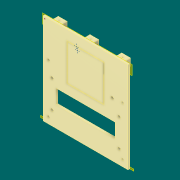
# Autodesk Inventor part: Front
Saved by Autodesk Inventor 2019 (Build 230136000, 136)
## iProperties
Created: 2025-01-01
Part Number: Front
Material: Nylon 6/6
Document SubType Name: Modeling
Designer: Familia CS
Density: 1.13 g/cm^3
Appearance: Nylon 6
Author: Familia CS
Autodesk Inventor part; units mm, degrees
ref_plane "YZ Plane" through (0, 0, 0) normal (1, 0, 0) x (0, 1, 0)
ref_plane "XZ Plane" through (0, 0, 0) normal (0, 1, 0) x (-1, 0, 0)
ref_plane "XY Plane" through (0, 0, 0) normal (0, 0, 1) x (1, 0, 0)
ref_plane "Work Plane1" through (0, 0, 0) normal (0, 0, 1) x (1, 0, 0)
sketch "Sketch1" plane through (0, 0, 0) normal (0, 0, 1) x (1, 0, 0)
  line L0 (5, 0) -> (86, 0) projected
  line L1 (86, -8) -> (86, 0) projected
  line L2 (5, 0) -> (5, -8) projected
  line L3 (43, 0) -> (43, -8) projected
  line L4 (53, -8) -> (53, 0) projected
  line L5 (86, 0) -> (76, 0)
  line L6 (76, 0) -> (76, -8)
  line L7 (76, -8) -> (86, -8)
  line L8 (86, -8) -> (86, 0)
  line L9 (5, 0) -> (15, 0)
  line L10 (15, 0) -> (15, -8)
  line L11 (15, -8) -> (5, -8)
  line L12 (5, -8) -> (5, 0)
  point P0 (0, 0)
  dimension "d0" = 10
  dimension "d1" = 8
  dimension "d3" = 10
  dimension "d4" = 8
  constraints: 16 end point, 4 parallel, 2 horizontal, 2 perpendicular
  measures "d0" distance of L7.end L6.end
  measures "d1" distance of L6.end L5.end
  measures "d3" distance of L10.end L11.end
  measures "d4" distance of L9.end L10.end
extrude "Extrusion1" add sketch "Sketch1" against normal blind 8
sketch "Sketch2" plane through (0, 0, 0) normal (0, 0, 1) x (1, 0, 0)
  line L0 (15, 0) -> (15, -8) projected
  line L1 (76, -8) -> (76, 0) projected
  line L2 (15, -8) -> (76, -8)
  line L3 (45.5, -8) -> (40.5, -8)
  line L4 (40.5, -8) -> (40.5, 0)
  line L5 (40.5, 0) -> (50.5, 0)
  line L6 (50.5, 0) -> (50.5, -8)
  point P0 (0, 0)
  dimension "d7" = 5
  dimension "d8" = 10
  constraints: 10 end point, 3 perpendicular, 2 point on line, 1 horizontal, 1 midpoint
  measures "d7" distance of L3.start L3.end
  measures "d8" distance of L4.end L5.end
extrude "Extrusion2" add sketch "Sketch2" against normal blind 8
sketch "Sketch3" plane through (76, -8, 0) normal (0, -1, 0) x (1, 0, 0)
  line L0 (10, -8) -> (0, -8) projected
  circle A0 centre (5, -4) radius 0.75
  line L1 (-25.5, -8) -> (-35.5, -8) projected
  circle A1 centre (-30.5, -4) radius 0.75
  line L2 (-61, -8) -> (-71, -8) projected
  circle A2 centre (-66, -4) radius 0.75
  point P0 (-76, 0)
  dimension "d12" = 1.5
  dimension "d14" = 1.5
  dimension "d16" = 1.5
  constraints: 3 centre point
  measures "d12" diameter of A0
  measures "d14" diameter of A1
  measures "d16" diameter of A2
extrude "Extrusion3" cut sketch "Sketch3" against normal blind 8
ref_plane "Work Plane2" through (93, -98, 0) normal (0, 0, 1) x (-1, 0, 0)
sketch "Sketch4" plane through (93, -98, 0) normal (0, 0, 1) x (-1, 0, 0)
  line L0 (10, 0) -> (10, -10) projected
  line L1 (85, 0) -> (85, -10) projected
  line L2 (95, 0) -> (0, 0) projected
  line L3 (10, 0) -> (20, 0)
  line L4 (20, 0) -> (20, -10)
  line L5 (20, -10) -> (10, -10)
  line L6 (10, -10) -> (10, 0)
  line L7 (85, -10) -> (75, -10)
  line L8 (75, -10) -> (75, 0)
  line L9 (75, 0) -> (85, 0)
  line L10 (85, 0) -> (85, -10)
  line L11 (75, 0) -> (20, 0)
  line L12 (47.5, -10) -> (52.5, -10)
  line L13 (52.5, -10) -> (52.5, 0)
  line L14 (52.5, 0) -> (42.5, 0)
  line L15 (42.5, 0) -> (42.5, -10)
  line L16 (42.5, -10) -> (47.5, -10)
  point P0 (93, -98)
  dimension "d19" = 10
  dimension "d20" = 10
  dimension "d21" = 10
  dimension "d22" = 10
  dimension "d24" = 5
  dimension "d25" = 10
  dimension "d26" = 10
  dimension "d27" = 10
  constraints: 28 end point, 4 parallel, 3 horizontal, 3 point on line, 2 perpendicular
  measures "d19" distance of L4.end L5.end
  measures "d20" distance of L3.end L4.end
  measures "d21" distance of L8.end L9.end
  measures "d22" distance of L7.end L8.end
  measures "d24" distance of L12.start L12.end
  measures "d25" distance of L12.end L13.end
  measures "d26" distance of L13.end L14.end
  measures "d27" distance of L14.end L15.end
extrude "Extrusion4" add sketch "Sketch4" against normal blind 8
sketch "Sketch5" plane through (73, -88, 0) normal (0, 1, 0) x (1, 0, 0)
  line L0 (10, 0) -> (0, 0) projected
  circle A0 centre (5, 4) radius 0.75
  line L1 (-22.5, 0) -> (-32.5, 0) projected
  circle A1 centre (-27.5, 4) radius 0.75
  line L2 (-55, 0) -> (-65, 0) projected
  circle A2 centre (-60, 4) radius 0.75
  point P0 (-73, 0)
  dimension "d31" = 1.5
  dimension "d33" = 1.5
  dimension "d35" = 1.5
  constraints: 3 centre point
  measures "d31" diameter of A0
  measures "d33" diameter of A1
  measures "d35" diameter of A2
extrude "Extrusion5" cut sketch "Sketch5" against normal blind 10
sketch "Sketch6" plane through (93, -98, 0) normal (0, 0, 1) x (1, 0, 0)
  line L0 (0, 0) -> (0, -2) projected
  line L1 (-93, 100) -> (-95, 100) projected
  line L2 (-95, 100) -> (0, 100)
  line L3 (0, 100) -> (0, -2)
  line L4 (0, -2) -> (-95, -2)
  line L5 (-95, -2) -> (-95, 100)
  circle A0 centre (-6, 50) radius 0.75 projected
  circle A1 centre (-6, 5) radius 0.75 projected
  circle A2 centre (-89, 5) radius 0.75 projected
  circle A3 centre (-89, 50) radius 0.75 projected
  point P0 (-93, 98)
  constraints: 8 end point, 2 parallel, 1 horizontal, 1 perpendicular
extrude "Extrusion6" add sketch "Sketch6" along normal blind 2
sketch "Sketch7" plane through (93, -98, 0) normal (0, 0, -1) x (-1, 0, 0)
  line L0 (42.5, 90) -> (52.5, 90) projected
  line L1 (47.5, 84) -> (80.5, 84)
  line L2 (80.5, 84) -> (80.5, 68)
  line L3 (80.5, 68) -> (14.5, 68)
  line L4 (14.5, 68) -> (14.5, 84)
  line L5 (14.5, 84) -> (47.5, 84)
  point P0 (93, 98)
  dimension "d41" = 33
  dimension "d42" = 16
  dimension "d43" = 66
  constraints: 10 end point, 4 perpendicular, 1 horizontal, 1 point on line
  measures "d41" distance of L1.start L1.end
  measures "d42" distance of L1.end L2.end
  measures "d43" distance of L2.end L3.end
extrude "Extrusion7" cut sketch "Sketch7" against normal blind 2
sketch "Sketch8" plane through (93, -98, 0) normal (0, 0, -1) x (-1, 0, 0)
  line L0 (14.5, 84) -> (80.5, 84) projected
  circle A0 centre (85.1, 86.9) radius 1.375
  circle A1 centre (9.9, 86.9) radius 1.375
  line L1 (80.5, 68) -> (14.5, 68) projected
  circle A2 centre (9.9, 65.1) radius 1.375
  circle A3 centre (85.1, 65.1) radius 1.375
  point P0 (93, 98)
  dimension "d50" = 2.75
  dimension "d54" = 2.75
  dimension "d61" = 2.75
  dimension "d64" = 2.75
  constraints: 4 centre point
  measures "d50" diameter of A0
  measures "d54" diameter of A1
  measures "d61" diameter of A2
  measures "d64" diameter of A3
extrude "Extrusion8" cut sketch "Sketch8" against normal blind 2
sketch "Sketch9" plane through (93, -98, 2) normal (0, 0, 1) x (1, 0, 0)
  line L0 (-88, 88.797) -> (-7.6952, 88.797)
  line L1 (-7.6952, 88.797) -> (-7.6952, 63.1475)
  line L2 (-7.6952, 63.1475) -> (-88, 63.1475)
  line L3 (-88, 63.1475) -> (-88, 88.797)
  point P0 (-93, 98)
  constraints: 8 end point, 2 parallel, 1 horizontal, 1 perpendicular
extrude "Extrusion9" add sketch "Sketch9" against normal blind 2
sketch "Sketch10" plane through (93, -98, 0) normal (0, 0, -1) x (-1, 0, 0)
  line L0 (42.5, 10) -> (52.5, 10) projected
  line L1 (47.5, 16) -> (14.5, 16)
  line L2 (14.5, 16) -> (14.5, 32)
  line L3 (14.5, 32) -> (80.5, 32)
  line L4 (80.5, 32) -> (80.5, 16)
  line L5 (80.5, 16) -> (47.5, 16)
  circle A0 centre (9.9, 13.1) radius 1.375
  circle A1 centre (85.1, 13.1) radius 1.375
  line L6 (47.5, 32) -> (47.5, 37.4)
  circle A2 centre (85.1, 34.9) radius 1.375
  circle A3 centre (9.9, 34.9) radius 1.375
  point P0 (93, 98)
  dimension "d70" = 33
  dimension "d71" = 16
  dimension "d72" = 66
  dimension "d73" = 16
  dimension "d74" = 33
  dimension "d80" = 2.75
  dimension "d83" = 2.75
  dimension "d84" = 5.4
  dimension "d89" = 2.75
  dimension "d92" = 2.75
  constraints: 12 end point, 4 centre point, 2 perpendicular, 1 midpoint, 1 point on line, 1 vertical
  measures "d70" distance of L1.start L1.end
  measures "d71" distance of L1.end L2.end
  measures "d72" distance of L2.end L3.end
  measures "d73" distance of L3.end L4.end
  measures "d74" distance of L4.end L1.start
  measures "d80" diameter of A0
  measures "d83" diameter of A1
  measures "d84" distance of L6.start L6.end
  measures "d89" diameter of A2
  measures "d92" diameter of A3
extrude "Extrusion10" cut sketch "Sketch10" against normal blind 2
sketch "Sketch11" plane through (93, -98, 0) normal (0, 0, -1) x (-1, 0, 0)
  circle A0 centre (85.1, 13.1) radius 1.375 projected
  line L0 (8.0573, 36.8158) -> (87.4686, 36.8158)
  line L1 (87.4686, 36.8158) -> (87.4686, 10.2199)
  line L2 (87.4686, 10.2199) -> (8.0573, 10.2199)
  line L3 (8.0573, 10.2199) -> (8.0573, 36.8158)
  point P0 (93, 98)
  constraints: 8 end point, 2 parallel, 1 horizontal, 1 perpendicular
extrude "Extrusion11" add sketch "Sketch11" against normal blind 2
sketch "Sketch12" plane through (93, -98, 0) normal (0, 0, -1) x (-1, 0, 0)
  line L0 (82.8776, 15.0849) -> (86.9969, 15.0849)
  line L1 (86.9969, 15.0849) -> (86.9969, 11.175)
  line L2 (86.9969, 11.175) -> (82.8776, 11.175)
  line L3 (82.8776, 11.175) -> (82.8776, 15.0849)
  point P0 (93, 98)
  constraints: 8 end point, 2 parallel, 1 horizontal, 1 perpendicular
extrude "Extrusion12" add sketch "Sketch12" against normal blind 2
sketch "Sketch13" plane through (93, -98, 0) normal (0, 0, -1) x (-1, 0, 0)
  line L0 (42.5, 10) -> (52.5, 10) projected
  circle A0 centre (85.1, 22.5) radius 2.75
  point P0 (93, 98)
  dimension "d104" = 5.5
  constraints: 1 centre point
  measures "d104" diameter of A0
extrude "Extrusion13" cut sketch "Sketch13" against normal blind 2
sketch "Sketch14" plane through (93, -98, 2) normal (0, 0, 1) x (1, 0, 0)
  line L0 (-88.4753, 26.414) -> (-81.2801, 26.414)
  line L1 (-81.2801, 26.414) -> (-81.2801, 18.3554)
  line L2 (-81.2801, 18.3554) -> (-88.4753, 18.3554)
  line L3 (-88.4753, 18.3554) -> (-88.4753, 26.414)
  point P0 (-93, 98)
  constraints: 8 end point, 2 parallel, 1 horizontal, 1 perpendicular
extrude "Extrusion14" add sketch "Sketch14" against normal blind 2
sketch "Sketch15" plane through (93, -98, 2) normal (0, 0, 1) x (1, 0, 0)
  point P0 (-93, 98)
sketch "Sketch16" plane through (93, -98, 0) normal (0, 0, -1) x (-1, 0, 0)
  line L0 (52.5, 90) -> (42.5, 90) projected
  circle A0 centre (9.9, 81.5) radius 1.5
  point P0 (93, 98)
  dimension "d118" = 3
  constraints: 1 centre point
  measures "d118" diameter of A0
extrude "Extrusion15" cut sketch "Sketch16" against normal blind 2
sketch "Sketch17" plane through (93, -98, 0) normal (0, 0, -1) x (-1, 0, 0)
  line L0 (7.2985, 84.1851) -> (12.7093, 84.1851)
  line L1 (12.7093, 84.1851) -> (12.7093, 78.544)
  line L2 (12.7093, 78.544) -> (7.2985, 78.544)
  line L3 (7.2985, 78.544) -> (7.2985, 84.1851)
  point P0 (93, 98)
  constraints: 8 end point, 2 parallel, 1 horizontal, 1 perpendicular
extrude "Extrusion16" add sketch "Sketch17" against normal blind 2
sketch "Sketch18" plane through (93, -98, 0) normal (0, 0, -1) x (-1, 0, 0)
  line L0 (42.5, 10) -> (52.5, 10) projected
  circle A0 centre (85.1, 18.5) radius 1.5
  point P0 (93, 98)
  dimension "d127" = 3
  constraints: 1 centre point
  measures "d127" diameter of A0
extrude "Extrusion17" cut sketch "Sketch18" against normal blind 2
sketch "Sketch19" plane through (93, -98, 0) normal (0, 0, -1) x (-1, 0, 0)
  line L0 (42.5, 10) -> (52.5, 10) projected
  circle A0 centre (9.9, 18.5) radius 1.5
  point P0 (93, 98)
  dimension "d134" = 3
  constraints: 1 centre point
  measures "d134" diameter of A0
extrude "Extrusion18" cut sketch "Sketch19" against normal blind 2
sketch "Sketch20" plane through (93, -98, 0) normal (0, 0, -1) x (-1, 0, 0)
  line L0 (6.951, 21.791) -> (88.5357, 21.791)
  line L1 (88.5357, 21.791) -> (88.5357, 14.1465)
  line L2 (88.5357, 14.1465) -> (6.951, 14.1465)
  line L3 (6.951, 14.1465) -> (6.951, 21.791)
  point P0 (93, 98)
  constraints: 8 end point, 2 parallel, 1 horizontal, 1 perpendicular
extrude "Extrusion19" add sketch "Sketch20" against normal blind 2
sketch "Sketch21" plane through (93, -98, 0) normal (0, 0, -1) x (-1, 0, 0)
  line L0 (42.5, 10) -> (52.5, 10) projected
  circle A0 centre (85.1, 13.5) radius 1.5
  circle A1 centre (9.9, 13.5) radius 1.5
  line L1 (47.5, 21) -> (80.5, 21)
  line L2 (80.5, 21) -> (80.5, 37)
  line L3 (80.5, 37) -> (14.5, 37)
  line L4 (14.5, 37) -> (14.5, 21)
  line L5 (14.5, 21) -> (47.5, 21)
  circle A2 centre (9.9, 44.5) radius 1.5
  circle A3 centre (85.1, 44.5) radius 1.5
  point P0 (93, 98)
  dimension "d143" = 3
  dimension "d147" = 3
  dimension "d150" = 33
  dimension "d151" = 16
  dimension "d152" = 66
  dimension "d157" = 3
  dimension "d161" = 3
  constraints: 10 end point, 4 centre point, 3 perpendicular, 1 horizontal, 1 vertical
  measures "d143" diameter of A0
  measures "d147" diameter of A1
  measures "d150" distance of L1.start L1.end
  measures "d151" distance of L1.end L2.end
  measures "d152" distance of L2.end L3.end
  measures "d157" diameter of A2
  measures "d161" diameter of A3
extrude "Extrusion20" cut sketch "Sketch21" against normal blind 2
sketch "Sketch22" plane through (93, -98, 0) normal (0, 0, -1) x (-1, 0, 0)
  line L0 (88.1, 50.9663) -> (90.0333, 50.9663)
  line L1 (90.0333, 50.9663) -> (90.0333, 48.9675)
  line L2 (90.0333, 48.9675) -> (88.1, 48.9675)
  line L3 (88.1, 48.9675) -> (88.1, 50.9663)
  line L4 (5.046, 50.7936) -> (6.9554, 50.7936)
  line L5 (6.9554, 50.7936) -> (6.9554, 48.9675)
  line L6 (6.9554, 48.9675) -> (5.046, 48.9675)
  line L7 (5.046, 48.9675) -> (5.046, 50.7936)
  point P0 (93, 98)
  constraints: 16 end point, 4 parallel, 2 horizontal, 2 perpendicular, 1 point on line
extrude "Extrusion21" add sketch "Sketch22" against normal blind 2
sketch "Sketch23" plane through (93, -98, 2) normal (0, 0, 1) x (1, 0, 0)
  point P0 (-93, 98)
  point P1 (-57.8, 88.8806)
  point P2 (-56.6, 85.3806)
  constraints: 2 other
sketch "Sketch24" plane through (93, -98, 2) normal (0, 0, 1) x (1, 0, 0)
  circle A0 centre (-89, 60) radius 0.75 projected
  point P0 (-93, 98)
extrude "Extrusion22" cut sketch "Sketch24" against normal blind 2
sketch "Sketch25" plane through (93, -98, 2) normal (0, 0, 1) x (1, 0, 0)
  circle A0 centre (-89, 60) radius 0.75 projected
  circle A1 centre (-89, 60) radius 1.25
  point P0 (-93, 98)
  dimension "d168" = 2.5
  constraints: 1 centre point, 1 coincident
  measures "d168" diameter of A1
extrude "Extrusion23" cut sketch "Sketch25" against normal blind 2
sketch "Sketch26" plane through (93, -98, 2) normal (0, 0, 1) x (1, 0, 0)
  circle A0 centre (-89, 5) radius 0.75 projected
  circle A1 centre (-89, 5) radius 1.25
  circle A2 centre (-6, 5) radius 0.75 projected
  circle A3 centre (-6, 5) radius 1.25
  point P0 (-93, 98)
  dimension "d171" = 2.5
  dimension "d172" = 2.5
  constraints: 2 centre point, 2 coincident
  measures "d171" diameter of A1
  measures "d172" diameter of A3
extrude "Extrusion24" cut sketch "Sketch26" against normal blind 2 contours A0 | A1 | A3
sketch "Sketch27" plane through (93, -98, 2) normal (0, 0, 1) x (1, 0, 0)
  point P0 (-93, 98)
sketch "Sketch28" plane through (93, -98, 2) normal (0, 0, 1) x (1, 0, 0)
  circle A0 centre (-6, 60) radius 0.75 projected
  circle A1 centre (-6, 60) radius 1.25
  point P0 (-93, 98)
  dimension "d175" = 2.5
  constraints: 1 centre point, 1 coincident
  measures "d175" diameter of A1
extrude "Extrusion25" cut sketch "Sketch28" against normal blind 2 contours A0 | A1
sketch "Sketch29" plane through (93, -98, 2) normal (0, 0, 1) x (1, 0, 0)
  circle A0 centre (-17.6001, 58.9999) radius 1.525 projected
  point P0 (-93, 98)
extrude "Extrusion26" cut sketch "Sketch29" against normal blind 2
sketch "Sketch30" plane through (93, -98, 2) normal (0, 0, 1) x (1, 0, 0)
  line L0 (-14.5, 37) -> (-80.5, 37) projected
  line L1 (-47.5, 37) -> (-47.5, 99.7686)
  line L2 (-27.5, 88.3843) -> (-67.5, 88.3843)
  line L3 (-67.5, 88.3843) -> (-67.5, 48.3843)
  line L4 (-67.5, 48.3843) -> (-27.5, 48.3843)
  line L5 (-27.5, 48.3843) -> (-27.5, 88.3843)
  line L6 (-27.5, 88.3843) -> (-67.5, 48.3843) construction
  line L7 (-67.5, 88.3843) -> (-27.5, 48.3843) construction
  line L8 (-26.5, 47.3843) -> (-68.5, 47.3843)
  line L9 (-68.5, 47.3843) -> (-68.5, 89.3843)
  line L10 (-68.5, 89.3843) -> (-26.5, 89.3843)
  line L11 (-26.5, 89.3843) -> (-26.5, 47.3843)
  point P0 (-93, 98)
  point P1 (-47.5, 68.3843)
  dimension "d180" = 40
  dimension "d181" = 40
  dimension "d182" = 1
  constraints: 22 end point, 4 midpoint, 4 parallel, 2 perpendicular, 1 horizontal, 1 vertical, 3 other
  measures "d180" distance of L4.end L3.end
  measures "d181" distance of L3.end L2.end
  measures "d182" distance between parallel lines of L4 L8
extrude "Extrusion27" cut sketch "Sketch30" against normal blind 0.5 contours L8 L9 L10 L1 L2 L3 L4 | L1 L4 L5 L2 L10 L11 L8
sketch "Sketch31" plane through (93, -98, 2) normal (0, 0, 1) x (1, 0, 0)
  line L0 (-27.5066, 88.3731) -> (-27.5066, 87.3731)
  line L1 (-26.5, 89.3843) -> (-26.5, 47.3843) projected
  line L2 (-27.5066, 87.3731) -> (-26.5, 87.3731)
  line L3 (-26.5, 87.3731) -> (-26.5, 76.3731)
  line L4 (-26.5, 76.3731) -> (-27.5066, 76.3731)
  line L5 (-27.5066, 76.3731) -> (-27.5066, 87.3731)
  point P0 (-93, 98)
  dimension "d185" = 1
  dimension "d186" = 11
  constraints: 10 end point, 2 parallel, 1 horizontal, 1 perpendicular, 1 point on line, 1 vertical
  measures "d185" distance of L0.start L0.end
  measures "d186" distance of L2.end L3.end
extrude "Extrusion28" cut sketch "Sketch31" against normal blind 1.5
sketch "Sketch32" plane through (93, -98, 0.5) normal (0, 0, 1) x (1, 0, 0)
  line L0 (-26.5, 76.3731) -> (-26.5, 47.3843) projected
  line L1 (-27.5066, 76.3731) -> (-27.5066, 87.3731) projected
  line L2 (-26.5, 76.3731) -> (-27.5066, 76.3731)
  line L3 (-27.5066, 76.3731) -> (-27.5066, 87.3731)
  line L4 (-27.5066, 87.3731) -> (-26.5, 87.3731)
  line L5 (-26.5, 87.3731) -> (-26.5, 76.3731)
  point P0 (-93, 98)
  constraints: 8 end point, 2 parallel, 1 horizontal, 1 perpendicular
extrude "Extrusion29" cut sketch "Sketch32" against normal blind 0.5
body "Solid1"
